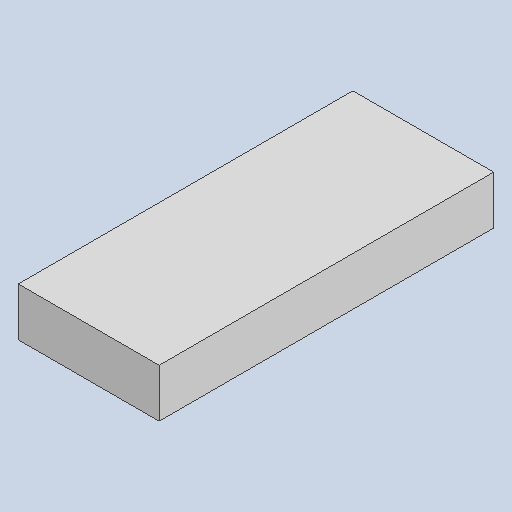
# Autodesk Inventor part: LiPo3000mAH
Saved by Autodesk Inventor 2025.1 (Build 291241000, 241)
## iProperties
Created: 2025-05-22
Part Number: LiPo3000mAH
Material: Generic
Document SubType Name: Modeling
Designer: User
Density: 1 g/cm^3
Appearance: Default
Author: User
Autodesk Inventor part; units mm, degrees
ref_plane "YZ Plane" through (0, 0, 0) normal (1, 0, 0) x (0, 1, 0)
ref_plane "XZ Plane" through (0, 0, 0) normal (0, 1, 0) x (-1, 0, 0)
ref_plane "XY Plane" through (0, 0, 0) normal (0, 0, 1) x (1, 0, 0)
sketch "Sketch1" plane through (0, 0, 0) normal (0, 0, 1) x (1, 0, 0)
  line L0 (-8.8755, 3.2604) -> (35.1245, 3.2604)
  line L1 (35.1245, 3.2604) -> (35.1245, -18.7396)
  line L2 (35.1245, -18.7396) -> (-8.8755, -18.7396)
  line L3 (-8.8755, -18.7396) -> (-8.8755, 3.2604)
  point P0 (0, 0)
  dimension "d0" = 44
  dimension "d1" = 22
  constraints: 8 end point, 2 parallel, 1 horizontal, 1 perpendicular
  measures "d0" distance of L1.end L2.end
  measures "d1" distance of L0.end L1.end
extrude "Extrusion1" add sketch "Sketch1" against normal blind 152
sketch "Sketch2" plane through (35.1245, -18.7396, 0) normal (1, 0, 0) x (0, 0, -1)
  line L0 (152, 22) -> (152, 0) projected
  line L1 (0, 22) -> (152, 22) projected
  line L2 (0, 0) -> (152, 0) projected
  line L3 (0, 0) -> (0, 22) projected
  point P0 (0, 18.7396)
extrude "Extrusion2" add sketch "Sketch2" along normal blind 20
body "Solid1"
